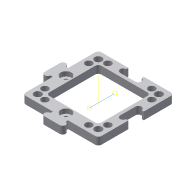
# Autodesk Inventor part: 10_Base_puzzle_v3
Saved by Autodesk Inventor 2022 (Build 260153000, 153)
## iProperties
Created: 2017-06-20
Part Number: 10_Base_puzzle_v3
Material: Generisch
Document SubType Name: Modeling
Designer: diederichbenedict
Density: 1 g/cm^3
Appearance: Weiß
Mass: 7.87446 g
Surface Area: 71.4468 cm^2
Volume: 7.87446 cm^3
d_part: 50,000 mm
d_o: 40,000 mm
d_i: 40,000 mm
Author: diederichbenedict
Autodesk Inventor part; units mm, degrees
ref_plane "YZ Plane" through (0, 0, 0) normal (1, 0, 0) x (0, 1, 0)
ref_plane "XZ Plane" through (0, 0, 0) normal (0, 1, 0) x (-1, 0, 0)
ref_plane "XY Plane" through (0, 0, 0) normal (0, 0, 1) x (1, 0, 0)
sketch "Skizze1" plane through (0, 0, 0) normal (0, 0, 1) x (1, 0, 0)
  line L0 (-17.25, 0) -> (-25, 0)
  line L1 (-25, 0) -> (-25, -23)
  line L2 (-23, -25) -> (0, -25)
  line L3 (0, -25) -> (0, -17.25)
  line L4 (-17.25, 0) -> (-17.25, -15.25)
  line L5 (-15.25, -17.25) -> (0, -17.25)
  arc A0 (-25, -23) -> (-23, -25) centre (-23, -23) ccw
  circle A1 centre (-20, -20) radius 2.45
  circle A2 centre (-20.8, -14.5) radius 2.3
  circle A3 centre (-14.5, -20.8) radius 2.3
  arc A4 (-17.25, -15.25) -> (-15.25, -17.25) centre (-15.25, -15.25) ccw
  circle A5 centre (-20, -20) radius 2.45
  circle A6 centre (-14.5, -20.8) radius 2.3
  circle A7 centre (-20.8, -14.5) radius 2.3
  line L6 (-41.8983, 0) -> (36.633, 0) construction
  line L7 (0, -35.5799) -> (0, 35.5799) construction
  point P0 (-25, -25)
  point P1 (-17.25, -17.25)
  dimension "d278" = 25
  dimension "d279" = 25
  dimension "d2" = 7.75
  dimension "d281" = 7.75
  dimension "d282" = 2
  dimension "d283" = 4.9
  dimension "d284" = 20
  dimension "d4" = 20
  dimension "d286" = 4.6
  dimension "d_hole" = 4.6
  dimension "d290" = 20.8
  dimension "d" = 20.8
  dimension "d292" = 2
  dimension "d313" = 6.3
  dimension "d314" = 6.3
  dimension "d330" = 0
  dimension "d331" = 0
  dimension "d332" = 0
  constraints: 12 end point, 8 centre point, 4 point on circle, 4 point on line, 4 tangent, 2 coincident, 2 collinear, 2 parallel, 1 horizontal, 1 perpendicular
  measures "d278" distance of L2.end point (-25, -25)
  measures "d279" distance of point (-25, -25) L0.end
  measures "d2" distance between parallel lines of L4 L1
  measures "d281" distance between parallel lines of L2 L5
  measures "d282" radius of A0
  measures "d283" diameter of A1
  measures "d284" distance from line of L0 A1.centre
  measures "d4" distance from line of L3 A1.centre
  measures "d286" diameter of A2
  measures "d_hole" diameter of A3
  measures "d290" distance from line of L0 A3.centre
  measures "d" distance from line of L3 A2.centre
  measures "d292" radius of A4
  measures "d313" horizontal distance of A2.centre A3.centre
  measures "d314" horizontal distance of A2.centre A3.centre
  measures "d330" radial gap between concentric circles of A1 A5
  measures "d331" radial gap between concentric circles of A3 A6
  measures "d332" radial gap between concentric circles of A2 A7
extrude "Extrusion1" add sketch "Skizze1" along normal blind 5
mirror "Mirror6" about plane through (-17.25, 0, 0) normal (0, 1, 0) of "Extrusion1"
mirror "Mirror7" about plane through (0, -25, 0) normal (1, 0, 0) of "Extrusion1", "Mirror6"
sketch "Sketch26" plane through (0, 0, 5) normal (0, 0, 1) x (1, 0, 0)
  line L0 (23, 25) -> (-23, 25) projected
  arc A0 (-23, 25) -> (-25, 23) centre (-23, 23) ccw projected
  line L1 (-25, -23) -> (-25, 23) projected
  arc A1 (-25, -23) -> (-23, -25) centre (-23, -23) ccw projected
  line L2 (-23, -25) -> (23, -25) projected
  arc A2 (23, -25) -> (25, -23) centre (23, -23) ccw projected
  line L3 (25, 23) -> (25, -23) projected
  arc A3 (25, 23) -> (23, 25) centre (23, 23) ccw projected
  line L4 (15.25, 17.25) -> (-15.25, 17.25) projected
  arc A4 (17.25, 15.25) -> (15.25, 17.25) centre (15.25, 15.25) ccw projected
  line L5 (17.25, 15.25) -> (17.25, -15.25) projected
  arc A5 (15.25, -17.25) -> (17.25, -15.25) centre (15.25, -15.25) ccw projected
  line L6 (-15.25, -17.25) -> (15.25, -17.25) projected
  arc A6 (-17.25, -15.25) -> (-15.25, -17.25) centre (-15.25, -15.25) ccw projected
  line L7 (-17.25, -15.25) -> (-17.25, 15.25) projected
  arc A7 (-15.25, 17.25) -> (-17.25, 15.25) centre (-15.25, 15.25) ccw projected
  line L8 (-25, -23) -> (-25, 23) projected
  line L9 (-28.55, -6.95) -> (-28.55, -6.95)
  line L10 (-30.5, -5) -> (-30.5, 5.1)
  line L11 (-28.55, 7.05) -> (-28.55, 7.05)
  line L12 (-25, 7) -> (-25, -7)
  line L13 (-26.1329, 5) -> (-25, 5)
  line L14 (-25, 5) -> (-25, -5)
  line L15 (-25, -5) -> (-26.1516, -5)
  line L16 (-26.5, -5) -> (-25, 5) construction
  line L17 (-26.5, 5) -> (-25, -5) construction
  arc A8 (-30.5, -5) -> (-28.55, -6.95) centre (-28.55, -5) ccw
  arc A9 (-28.55, -6.95) -> (-26.641, -5.398) centre (-28.55, -5) ccw
  arc A10 (-28.55, 7.05) -> (-30.5, 5.1) centre (-28.55, 5.1) ccw
  arc A11 (-26.6262, 5.4184) -> (-28.55, 7.05) centre (-28.55, 5.1) ccw
  arc A12 (-26.1516, -5) -> (-26.641, -5.398) centre (-26.1516, -5.5) ccw
  arc A13 (-26.6262, 5.4184) -> (-26.1329, 5) centre (-26.1329, 5.5) ccw
  point P0 (0, 0)
  point P1 (-25.75, 0)
  point P2 (-25, 0)
  dimension "d293" = 5.5
  dimension "d294" = 14
  dimension "d296" = 10
  dimension "d297" = 1.5
  dimension "d300" = 1.95
  dimension "d301" = 0.5
  dimension "d357" = 5
  constraints: 18 end point, 12 point on circle, 10 tangent, 6 centre point, 4 equal radius, 4 midpoint, 3 parallel, 3 point on line, 2 coincident, 1 horizontal, 1 perpendicular
  measures "d293" distance between parallel lines of L1 L10
  measures "d294" distance between parallel lines of L9 L11
  measures "d296" distance of L16.start L17.start
  measures "d297" distance of L17.start L13.end
  measures "d300" radius of A8
  measures "d301" radius of A12
  measures "d357" distance from line of point (-25, 0) L13
extrude "Extrusion13" add sketch "Sketch26" against normal up to surface (5 mm away) contours L1 L15 A12 A9 A8 L10 A10 A11 A13 L13
sketch "Sketch28" plane through (0, 0, 5) normal (0, 0, 1) x (1, 0, 0)
  line L0 (-41.9326, 0) -> (36.8388, 0) construction
  line L1 (23, 25) -> (-23, 25) projected
  arc A0 (-23, 25) -> (-25, 23) centre (-23, 23) ccw projected
  line L2 (-25, 5) -> (-25, 23) projected
  line L3 (-26.1329, 5) -> (-25, 5) projected
  arc A1 (-26.6262, 5.4184) -> (-26.1329, 5) centre (-26.1329, 5.5) ccw projected
  arc A2 (-26.6262, 5.4184) -> (-30.5, 5.1) centre (-28.55, 5.1) ccw projected
  line L4 (-30.5, -5) -> (-30.5, 5.1) projected
  arc A3 (-30.5, -5) -> (-26.641, -5.398) centre (-28.55, -5) ccw projected
  arc A4 (-26.1516, -5) -> (-26.641, -5.398) centre (-26.1516, -5.5) ccw projected
  line L5 (-25, -5) -> (-26.1516, -5) projected
  line L6 (-25, -23) -> (-25, -5) projected
  arc A5 (-25, -23) -> (-23, -25) centre (-23, -23) ccw projected
  line L7 (-23, -25) -> (23, -25) projected
  arc A6 (23, -25) -> (25, -23) centre (23, -23) ccw projected
  line L8 (25, 23) -> (25, -23) projected
  arc A7 (25, 23) -> (23, 25) centre (23, 23) ccw projected
  circle A8 centre (20, 20) radius 2.45 projected
  circle A9 centre (14.5, 20.8) radius 2.3 projected
  circle A10 centre (20.8, 14.5) radius 2.3 projected
  circle A11 centre (20, -20) radius 2.45 projected
  circle A12 centre (14.5, -20.8) radius 2.3 projected
  circle A13 centre (20.8, -14.5) radius 2.3 projected
  circle A14 centre (-20, 20) radius 2.45 projected
  circle A15 centre (-14.5, 20.8) radius 2.3 projected
  circle A16 centre (-20.8, 14.5) radius 2.3 projected
  circle A17 centre (-20.8, -14.5) radius 2.3 projected
  circle A18 centre (-14.5, -20.8) radius 2.3 projected
  circle A19 centre (-20, -20) radius 2.45 projected
  line L9 (15.25, 17.25) -> (-15.25, 17.25) projected
  arc A20 (17.25, 15.25) -> (15.25, 17.25) centre (15.25, 15.25) ccw projected
  line L10 (17.25, 15.25) -> (17.25, -15.25) projected
  arc A21 (15.25, -17.25) -> (17.25, -15.25) centre (15.25, -15.25) ccw projected
  line L11 (-15.25, -17.25) -> (15.25, -17.25) projected
  arc A22 (-17.25, -15.25) -> (-15.25, -17.25) centre (-15.25, -15.25) ccw projected
  line L12 (-17.25, -15.25) -> (-17.25, 15.25) projected
  arc A23 (-15.25, 17.25) -> (-17.25, 15.25) centre (-15.25, 15.25) ccw projected
  line L13 (-25, 5) -> (-24.4142, 5)
  line L14 (-24.4142, 5) -> (-24.4142, -5)
  line L15 (-24.4142, -5) -> (-25, -5)
  line L16 (-25, -5) -> (-25, 5)
  line L17 (-26.1329, 5) -> (-25, 5) projected
  line L18 (-25, 5) -> (-26.1329, 5)
  line L19 (-30.5, -5) -> (-30.5, 5.1) projected
  line L20 (-30.5, 5.1) -> (-30.5, -5)
  line L21 (-25, -5) -> (-25, -23) projected
  line L22 (-25, -5) -> (-26.1516, -5)
  line L23 (-25, -5) -> (-26.1516, -5) projected
  arc A24 (-26.1516, -5) -> (-26.641, -5.398) centre (-26.1516, -5.5) ccw projected
  arc A25 (-26.1516, -5) -> (-26.641, -5.398) centre (-26.1516, -5.5) ccw
  arc A26 (-30.5, -5) -> (-26.641, -5.398) centre (-28.55, -5) ccw
  arc A27 (-26.6262, 5.4184) -> (-26.1329, 5) centre (-26.1329, 5.5) ccw projected
  arc A28 (-26.6262, 5.4184) -> (-30.5, 5.1) centre (-28.55, 5.1) ccw
  arc A29 (-26.6262, 5.4184) -> (-26.1329, 5) centre (-26.1329, 5.5) ccw
  line L24 (25, 5) -> (25.5858, 5)
  line L25 (25.5858, 5) -> (25.5858, -5)
  line L26 (25.5858, -5) -> (25, -5)
  line L27 (25, -5) -> (25, 5)
  line L28 (25, 5) -> (23.8671, 5)
  line L29 (19.5, 5.1) -> (19.5, -5)
  line L30 (25, -5) -> (23.8484, -5)
  arc A30 (23.8484, -5) -> (23.359, -5.398) centre (23.8484, -5.5) ccw
  arc A31 (19.5, -5) -> (23.359, -5.398) centre (21.45, -5) ccw
  arc A32 (23.3738, 5.4184) -> (19.5, 5.1) centre (21.45, 5.1) ccw
  arc A33 (23.3738, 5.4184) -> (23.8671, 5) centre (23.8671, 5.5) ccw
  line L31 (25, 23) -> (25, -23) projected
  arc A34 (19.4, -5) -> (23.4629, -5.3883) centre (21.45, -5) ccw
  line L32 (19.4, -5) -> (19.4, 5.1)
  arc A35 (23.4725, 5.4347) -> (19.4, 5.1) centre (21.45, 5.1) ccw
  arc A36 (23.4725, 5.4347) -> (23.8671, 5.1) centre (23.8671, 5.5) ccw
  line L33 (23.8671, 5.1) -> (25, 5.1)
  line L34 (25, 5.1) -> (25, -5.1123)
  line L35 (25, -23) -> (25, 23) projected
  arc A37 (23.8687, -5.1123) -> (23.4629, -5.3883) centre (23.8044, -5.4541) ccw
  line L36 (25, -5.1123) -> (23.8687, -5.1123)
  point P0 (25, -5.1123)
  dimension "d358" = 5.5
  dimension "d359" = 0.1
  constraints: 36 end point, 28 point on circle, 12 centre point, 7 tangent, 5 equal length, 5 horizontal, 3 point on line, 2 concentric, 2 perpendicular, 4 other
  measures "d358" distance between parallel lines of L27 L29
  measures "d359" radial gap between concentric circles of A32 A35
extrude "Extrusion14" cut sketch "Sketch28" against normal blind 10 contours L8 L28 A33 A32 L29 A31 A30 L30 L36 A37 A34 L32 A35 A36 L33 | L8 L30 A30 A31 L29 A32 A33 L28
pattern_circular "Circular Pattern6" count 2 over 90 about axis through (0, 0, 5) along (0, 0, 1) of "Extrusion14", "Extrusion13"
sketch "Sketch29" plane through (0, 0, 5) normal (0, 0, 1) x (1, 0, 0)
  line L0 (-5.1, 25) -> (-23, 25) projected
  arc A0 (-23, 25) -> (-25, 23) centre (-23, 23) ccw projected
  line L1 (-25, 5) -> (-25, 23) projected
  line L2 (-26.1329, 5) -> (-25, 5) projected
  arc A1 (-26.6262, 5.4184) -> (-26.1329, 5) centre (-26.1329, 5.5) ccw projected
  arc A2 (-26.6262, 5.4184) -> (-30.5, 5.1) centre (-28.55, 5.1) ccw projected
  line L3 (-30.5, -5) -> (-30.5, 5.1) projected
  arc A3 (-30.5, -5) -> (-26.641, -5.398) centre (-28.55, -5) ccw projected
  arc A4 (-26.1516, -5) -> (-26.641, -5.398) centre (-26.1516, -5.5) ccw projected
  line L4 (-25, -5) -> (-26.1516, -5) projected
  line L5 (-25, -23) -> (-25, -5) projected
  arc A5 (-25, -23) -> (-23, -25) centre (-23, -23) ccw projected
  line L6 (-23, -25) -> (-5, -25) projected
  line L7 (-5, -26.1329) -> (-5, -25) projected
  arc A6 (-5.4184, -26.6262) -> (-5, -26.1329) centre (-5.5, -26.1329) ccw projected
  arc A7 (-5.4184, -26.6262) -> (-5.1, -30.5) centre (-5.1, -28.55) ccw projected
  line L8 (5, -30.5) -> (-5.1, -30.5) projected
  arc A8 (5, -30.5) -> (5.398, -26.641) centre (5, -28.55) ccw projected
  arc A9 (5, -26.1516) -> (5.398, -26.641) centre (5.5, -26.1516) ccw projected
  line L9 (5, -25) -> (5, -26.1516) projected
  line L10 (5, -25) -> (23, -25) projected
  arc A10 (23, -25) -> (25, -23) centre (23, -23) ccw projected
  line L11 (25, -5.1123) -> (25, -23) projected
  arc A11 (25, 23) -> (23, 25) centre (23, 23) ccw projected
  line L12 (15.25, 17.25) -> (-15.25, 17.25) projected
  arc A12 (17.25, 15.25) -> (15.25, 17.25) centre (15.25, 15.25) ccw projected
  line L13 (17.25, 15.25) -> (17.25, -15.25) projected
  arc A13 (15.25, -17.25) -> (17.25, -15.25) centre (15.25, -15.25) ccw projected
  line L14 (-15.25, -17.25) -> (15.25, -17.25) projected
  arc A14 (-17.25, -15.25) -> (-15.25, -17.25) centre (-15.25, -15.25) ccw projected
  line L15 (-17.25, -15.25) -> (-17.25, 15.25) projected
  arc A15 (-15.25, 17.25) -> (-17.25, 15.25) centre (-15.25, 15.25) ccw projected
  circle A16 centre (-21.36, 0) radius 3.89
  circle A17 centre (0, -21.36) radius 2.9259
  line L16 (-41.8983, 0) -> (36.633, 0) construction
  line L17 (0, -41.8983) -> (0, 36.633) construction
  line L18 (5.1123, 25) -> (5.1123, 23.8687) projected
  arc A18 (5.1123, 23.8687) -> (5.3883, 23.4629) centre (5.4541, 23.8044) ccw projected
  arc A19 (5, 19.4) -> (5.3883, 23.4629) centre (5, 21.45) ccw projected
  line L19 (5, 19.4) -> (-5.1, 19.4) projected
  arc A20 (-5.4347, 23.4725) -> (-5.1, 19.4) centre (-5.1, 21.45) ccw projected
  arc A21 (-5.4347, 23.4725) -> (-5.1, 23.8671) centre (-5.5, 23.8671) ccw projected
  line L20 (-5.1, 23.8671) -> (-5.1, 25) projected
  line L21 (25, -5.1123) -> (23.8687, -5.1123) projected
  arc A22 (23.8687, -5.1123) -> (23.4629, -5.3883) centre (23.8044, -5.4541) ccw projected
  arc A23 (19.4, -5) -> (23.4629, -5.3883) centre (21.45, -5) ccw projected
  line L22 (19.4, -5) -> (19.4, 5.1) projected
  arc A24 (23.4725, 5.4347) -> (19.4, 5.1) centre (21.45, 5.1) ccw projected
  arc A25 (23.4725, 5.4347) -> (23.8671, 5.1) centre (23.8671, 5.5) ccw projected
  line L23 (23.8671, 5.1) -> (25, 5.1) projected
  line L24 (25, 23) -> (25, 5.1) projected
  line L25 (23, 25) -> (5.1123, 25) projected
  point P0 (0, 0)
  dimension "d319" = 7.78
  dimension "d320" = 4.11
  dimension "d322" = 4.11
  constraints: 2 centre point, 2 point on line, 1 coincident
  measures "d319" diameter of A16
  measures "d320" distance from line of A16.centre L15
  measures "d322" distance from line of L14 A17.centre
hole "Hole7" at (-21.36, 0, 5) at (0, -21.36, 5) direction (0, 0, -1) diameter 3.2 end through all counterbore diameter 7 counterbore depth 3
equation "\"d_i\" = 40"
equation "\"d_o\" = 40"
equation "\"d_part\" = 50"
equation "\"d6\" = 0"
equation "\"d7\" = 0"
equation "\"d8\" = 0"
equation "\"d9\" = 0"
equation "\"d13\" = 0"
equation "\"d14\" = 0"
equation "\"d20\" = 0"
equation "\"d21\" = 0"
equation "\"d22\" = 0"
equation "\"d23\" = 0"
equation "\"d24\" = 0"
equation "\"d25\" = 3"
equation "\"d26\" = 0"
equation "\"d27\" = 0"
equation "\"d28\" = 0"
equation "\"d29\" = 0"
equation "\"d30\" = 0"
equation "\"d31\" = 0"
equation "\"d32\" = 0"
equation "\"d33\" = 0"
equation "\"d34\" = 0"
equation "\"d46\" = 0"
equation "\"d47\" = 0"
equation "\"d48\" = 0"
equation "\"d50\" = 0"
equation "\"d51\" = 0"
equation "\"d52\" = 0"
equation "\"d53\" = 0"
equation "\"d54\" = 0"
equation "\"d55\" = 0"
equation "\"d56\" = 0"
equation "\"d57\" = 0"
equation "\"d58\" = 0"
equation "\"d59\" = 0"
equation "\"magnet_offset\" = 0"
equation "\"screw_offset\" = 0"
equation "\"mal_puzzle_offset\" = 0"
equation "\"fem_puzzle_offset\" = 0"
